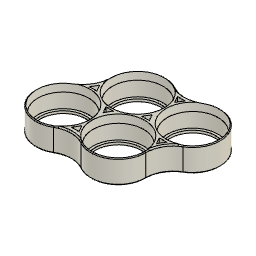
21700 hex cell holder v4 (Autodesk Fusion 360 design; units mm, degrees)
Autodesk Fusion 360 part; units mm, degrees
sketch "Sketch1" plane through (0, 0, 0) normal (0, 0, 1) x (1, 0, 0)
  circle A0 centre (0, 0) radius 10.55
  circle A1 centre (-22.7, -0.165603) radius 10.55
  circle A2 centre (-11.206589, -19.740881) radius 10.55
  circle A3 centre (0, 0) radius 11.35
  circle A4 centre (-22.7, -0.165603) radius 11.35
  circle A5 centre (-11.206589, -19.740881) radius 11.35
  arc A6 (5.746405, -9.787815) -> (0.14311, -19.658256) centre (11.49281, -19.575631) ccw
  circle A7 centre (-33.906589, -19.906483) radius 10.55
  circle A8 centre (-33.906589, -19.906483) radius 11.35
  arc A9 (-16.809883, -29.611321) -> (-28.159883, -29.694122) centre (-22.413178, -39.481761) ccw
  arc A10 (-39.652994, -10.118668) -> (-34.049699, -0.248228) centre (-45.399399, -0.330852) ccw
  arc A11 (-17.096706, 9.704838) -> (-5.746706, 9.787639) centre (-11.493411, 19.575278) ccw
  dimension "d1" = 21.1
  dimension "d3" = 21.1
  dimension "d6" = 21.1
  dimension "d7" = 22.7
  dimension "d9" = 22.7
  dimension "d10" = 22.7
  dimension "d14" = 22.7
  dimension "d15" = 22.7
  dimension "d16" = 22.7
  dimension "d17" = 22.7
  dimension "d18" = 21.1
  dimension "d19" = 22.7
  dimension "d20" = 22.7
  dimension "d21" = 22.7
  dimension "d22" = 22.7
  dimension "d23" = 22.7
  dimension "d24" = 22.7
  constraint coincident A0.centre A3.centre
  constraint concentric A1 A4
  constraint concentric A2 A5
  constraint tangent A5 A6
  constraint tangent A3 A6
  constraint concentric A7 A8
  constraint tangent A8 A9
  constraint tangent A5 A9
  constraint tangent A4 A10
  constraint tangent A8 A10
  constraint tangent A3 A11
  constraint tangent A4 A11
  measures "d1" diameter of A0
  measures "d3" diameter of A1
  measures "d6" diameter of A2
  measures "d14" diameter of A3
  measures "d15" diameter of A4
  measures "d16" diameter of A5
  measures "d17" diameter of A6
  measures "d18" diameter of A7
  measures "d19" diameter of A8
  measures "d22" diameter of A9
  measures "d23" diameter of A10
  measures "d24" diameter of A11
extrude "Extrude1" add sketch "Sketch1" along normal blind 10 contours A3 | A3 A4 A11 | A3 A5 A6 | A4 | A3 A4 A5 | A5 | A4 A5 A8 | A4 A8 A10 | A8 | A5 A8 A9 picked at (4.688349, 9.725973) picked at (-11.680435, 6.454432) picked at (0.381693, -13.593133) picked at (-13.356431, 5.244811) picked at (-11.022833, -6.172088) picked at (-21.247696, -15.772237) picked at (-22.887024, -13.286448) picked at (-33.71571, -7.288609) picked at (-24.56302, -14.49607) picked at (-22.229422, -25.912969)
sketch "Sketch2" plane through (0, 0, 0) normal (0, 0, -1) x (1, 0, 0)
  circle A0 centre (-11.206589, 19.740881) radius 10.55
  circle A1 centre (-22.7, 0.165603) radius 10.55
  circle A2 centre (-33.906589, 19.906483) radius 10.55
  circle A3 centre (0, 0) radius 10.55
  arc A4 (-34.049699, 0.248228) -> (-17.096706, -9.704838) centre (-22.7, 0.165603) ccw
  arc A5 (-5.746706, -9.787639) -> (-17.096706, -9.704838) centre (-11.493411, -19.575278) ccw
  arc A6 (-5.746706, -9.787639) -> (5.746405, 9.787815) centre (0, 0) ccw
  arc A7 (0.14311, 19.658256) -> (5.746405, 9.787815) centre (11.49281, 19.575631) ccw
  arc A8 (0.14311, 19.658256) -> (-16.809883, 29.611321) centre (-11.206589, 19.740881) ccw
  arc A9 (-28.159883, 29.694122) -> (-16.809883, 29.611321) centre (-22.413178, 39.481761) ccw
  arc A10 (-28.159883, 29.694122) -> (-39.652994, 10.118668) centre (-33.906589, 19.906483) ccw
  arc A11 (-34.049699, 0.248228) -> (-39.652994, 10.118668) centre (-45.399399, 0.330852) ccw
  circle A12 centre (-33.906589, 19.906483) radius 9.5
  circle A13 centre (-11.206589, 19.740881) radius 9.5
  circle A14 centre (-22.7, 0.165603) radius 9.5
  circle A15 centre (0, 0) radius 9.5
  dimension "d27" = 19
  dimension "d28" = 19
  dimension "d29" = 19
  dimension "d30" = 19
  constraint concentric A2 A12
  constraint concentric A0 A13
  constraint concentric A1 A14
  constraint coincident A3.centre A6.centre
  measures "d27" diameter of A12
  measures "d28" diameter of A13
  measures "d29" diameter of A14
  measures "d30" diameter of A15
extrude "Extrude2" add sketch "Sketch2" against normal blind 1 contours A0 | A1 | A2 | A3 picked at (-1.045867, 19.216749) picked at (-12.539278, -0.358529) picked at (-23.781236, 18.910384) picked at (10.160722, -0.524132)
sketch "Sketch4" plane through (0, 0, 0) normal (0, 0, -1) x (1, 0, 0)
  circle A0 centre (-33.906589, 19.906483) radius 9.5
  circle A1 centre (0, 0) radius 9.5
  circle A2 centre (-22.7, 0.165603) radius 9.5
  circle A3 centre (-11.206589, 19.740881) radius 9.5
  arc A4 (-34.049699, 0.248228) -> (-17.096706, -9.704838) centre (-22.7, 0.165603) ccw
  arc A5 (-5.746706, -9.787639) -> (-17.096706, -9.704838) centre (-11.493411, -19.575278) ccw
  arc A6 (-5.746706, -9.787639) -> (5.746405, 9.787815) centre (0, 0) ccw
  arc A7 (0.14311, 19.658256) -> (5.746405, 9.787815) centre (11.49281, 19.575631) ccw
  arc A8 (0.14311, 19.658256) -> (-16.809883, 29.611321) centre (-11.206589, 19.740881) ccw
  arc A9 (-28.159883, 29.694122) -> (-16.809883, 29.611321) centre (-22.413178, 39.481761) ccw
  arc A10 (-28.159883, 29.694122) -> (-39.652994, 10.118668) centre (-33.906589, 19.906483) ccw
  arc A11 (-34.049699, 0.248228) -> (-39.652994, 10.118668) centre (-45.399399, 0.330852) ccw
  line L0 (-23.97716, 26.406689) -> (-20.862148, 26.406689)
  line L1 (-20.862148, 26.406689) -> (-22.386515, 23.755616)
  line L2 (-22.386515, 23.755616) -> (-23.97716, 26.406689)
  line L3 (-22.651623, 14.543134) -> (-21.060979, 11.89206)
  line L4 (-24.17599, 11.89206) -> (-22.651623, 14.543134)
  line L5 (-21.060979, 11.89206) -> (-24.17599, 11.89206)
  line L6 (-12.975203, -6.665456) -> (-11.450836, -4.014382)
  line L7 (-9.860192, -6.665456) -> (-12.975203, -6.665456)
  line L8 (-11.450836, -4.014382) -> (-9.860192, -6.665456)
  line L9 (-10.191576, 7.849173) -> (-11.715943, 5.198099)
  line L10 (-13.306588, 7.849173) -> (-10.191576, 7.849173)
  line L11 (-11.715943, 5.198099) -> (-13.306588, 7.849173)
  line L12 (-33.26834, 5.472672) -> (-34.858984, 8.123746)
  line L13 (-34.858984, 8.123746) -> (-31.743972, 8.123746)
  line L14 (-31.743972, 8.123746) -> (-33.26834, 5.472672)
  line L15 (-0.394236, 14.64837) -> (1.196409, 11.997296)
  line L16 (1.196409, 11.997296) -> (-1.918603, 11.997296)
  line L17 (-1.918603, 11.997296) -> (-0.394236, 14.64837)
  constraint horizontal L0
  constraint horizontal L10
extrude "Extrude4" cut sketch "Sketch4" against normal through all contours L0 L1 L2 | L3 L4 L5 | L6 L7 L8 | L9 L10 L11 | L12 L13 L14 | L15 L16 L17 picked at (-22.408608, 25.522998) picked at (-22.629531, 12.775752) picked at (-11.428744, -5.781765) picked at (-11.738036, 6.965482) picked at (-33.290432, 7.240055) picked at (-0.372143, 12.880988)
chamfer "Chamfer1" distance 0.5 distance2 3 4 edges at (-9.836053, 3.815043, 10) (-32.536053, 3.64944, 10) (-43.742642, -16.09144, 10) (-21.042642, -15.925838, 10) measured on face at (-10.208113, -6.3301, 10) measured on face at (-10.208113, -6.3301, 10) measured on face at (-10.208113, -6.3301, 10) measured on face at (-10.208113, -6.3301, 10)
chamfer "Chamfer2" distance 0.5 angle 45 8 edges at (-11.410612, 8.22558, 10) (-28.446405, 9.622213, 10) (-35.528958, -5.934147, 10) (-43.694316, -25.653038, 10) (-22.495977, -28.132063, 10) (-5.460184, -29.528696, 10) (1.622369, -13.972337, 10) (9.787727, 5.746555, 10)
chamfer "Chamfer3" distance 0.5 angle 45 8 edges at (-11.410612, 8.22558, 0) (-28.446405, 9.622213, 0) (-35.528958, -5.934147, 0) (-43.694316, -25.653038, 0) (-22.495977, -28.132063, 0) (-5.460184, -29.528696, 0) (1.622369, -13.972337, 0) (9.787727, 5.746555, 0)
